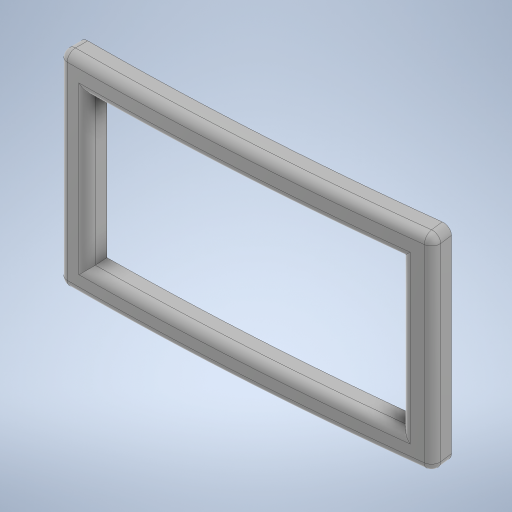
# Autodesk Inventor part: buckle
Saved by Autodesk Inventor 2024 (Build 280153000, 153)
## iProperties
Created: 2025-11-15
Part Number: buckle
Material: PC/ABS Plastic
Document SubType Name: Modeling
Designer: garys
Density: 1.1 g/cm^3
Appearance: Smooth - White
Author: garys
Autodesk Inventor part; units mm, degrees
ref_plane "YZ Plane" through (0, 0, 0) normal (1, 0, 0) x (0, 1, 0)
ref_plane "XZ Plane" through (0, 0, 0) normal (0, 1, 0) x (-1, 0, 0)
sketch "Sketch1" plane through (0, 0, 0) normal (1, 0, 0) x (0, 1, 0)
  line L0 (0, 0) -> (12.7, 0)
  line L1 (12.7, 0) -> (12.7, -1.27)
  line L2 (12.7, -1.27) -> (0, -1.27)
  line L3 (0, -1.27) -> (0, 0)
  line L4 (0, -1.27) -> (0, -179.07)
  line L5 (0, -179.07) -> (11.2239, -179.07)
  dimension "d0" = 12.7
  dimension "d1" = 1.27
  dimension "d2" = 177.8
  constraints: 12 end point, 2 parallel, 2 perpendicular, 1 horizontal, 1 vertical
  measures "d0" distance of L1.end L2.end
  measures "d1" distance of L0.end L1.end
  measures "d2" distance of L2.end L4.end
revolve "Revolution1" add sketch "Sketch1" angle 7 about axis through (0, 0, -179.07) along (0, 1, 0)
ref_plane "Work Plane1" through (21.6684, 0, -2.5953) normal (0.0610485, 0, 0.9981348) x (0, 1, 0)
sketch "Sketch3" plane through (21.6684, 0, -2.5953) normal (0.0610485, 0, 0.9981348) x (0, 1, 0)
  line L0 (10.9297, 1.7542) -> (1.6736, 1.7542)
  line L1 (1.6736, 1.7542) -> (1.6736, 20.0274)
  line L2 (1.6736, 20.0274) -> (10.9297, 20.0274)
  line L3 (10.9297, 20.0274) -> (10.9297, 1.7542)
  point P0 (0, 21.7864)
  constraints: 8 end point, 2 parallel, 1 horizontal, 1 perpendicular
extrude "Extrusion2" cut sketch "Sketch3" along normal blind 25.4
fillet "Fillet1" radius 0.508 12 edges at (0, 6.35, 0) (10.932, 12.7, -0.334) (21.8231, 6.35, -1.3348) (10.932, 0, -0.334) (10.8956, 1.6736, -0.3318) (20.0011, 6.3017, -1.1205) (1.7618, 6.3017, -0.0087) (10.8956, 10.9297, -0.3318) (21.7458, 12.7, -1.965) (0, 12.7, -0.635) (21.7458, 0, -1.965) (0, 0, -0.635)
body "Solid1"
